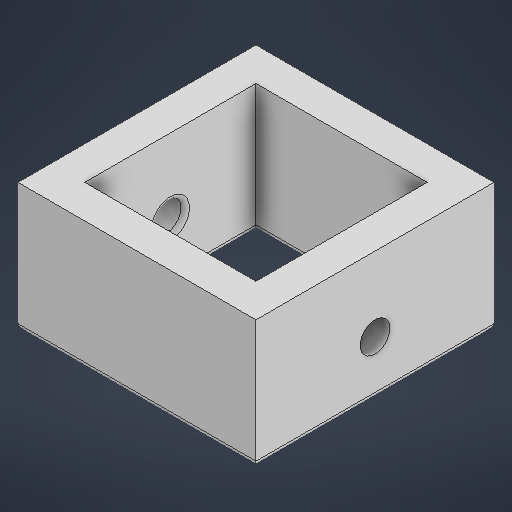
# Autodesk Inventor part: TestSujetaPerfil
Saved by Autodesk Inventor 2026.1 (Build 301233020, 233B)
## iProperties
Created: 2025-10-19
Part Number: TestSujetaPerfil
Material: Generic
Document SubType Name: Modeling
Designer: tito.luyo
Density: 1 g/cm^3
Appearance: Default
Author: tito.luyo
Autodesk Inventor part; units mm, degrees
ref_plane "YZ Plane" through (0, 0, 0) normal (1, 0, 0) x (0, 1, 0)
ref_plane "XZ Plane" through (0, 0, 0) normal (0, 1, 0) x (-1, 0, 0)
ref_plane "XY Plane" through (0, 0, 0) normal (0, 0, 1) x (1, 0, 0)
sketch "Sketch1" plane through (0, 0, 0) normal (0, 1, 0) x (-1, 0, 0)
  line L0 (0, 0) -> (28, 0)
  line L1 (28, 0) -> (28, -28)
  line L2 (28, -28) -> (0, -28)
  line L3 (0, -28) -> (0, 0)
  line L4 (24.075, -3.925) -> (3.925, -3.925)
  line L5 (3.925, -3.925) -> (3.925, -24.075)
  line L6 (3.925, -24.075) -> (24.075, -24.075)
  line L7 (24.075, -24.075) -> (24.075, -3.925)
  line L8 (24.075, -3.925) -> (3.925, -24.075) construction
  line L9 (3.925, -3.925) -> (24.075, -24.075) construction
  line L10 (0, 0) -> (28, -28) construction
  line L11 (28, 0) -> (0, -28) construction
  point P0 (14, -14)
  dimension "d0" = 28
  dimension "d1" = 28
  dimension "d2" = 20.15
  dimension "d3" = 20.15
  constraints: 24 end point, 4 parallel, 3 midpoint, 2 horizontal, 2 perpendicular
  measures "d0" distance of L1.end L2.end
  measures "d1" distance of L0.end L1.end
  measures "d2" distance of L6.end L5.end
  measures "d3" distance of L5.end L4.end
extrude "Extrusion1" add sketch "Sketch1" along normal blind 15
fillet "Fillet1" radius 0.6 8 edges at (-14, 0, -3.925) (-24.075, 0, -14) (-14, 0, -24.075) (-3.925, 0, -14) (-14, 0, 0) (-28, 0, -14) (-14, 0, -28) (0, 0, -14)
sketch "Sketch2" plane through (-28, 15, -28) normal (-1, 0, 0) x (0, 0, 1)
  circle A0 centre (14, -8.7403) radius 1.75
  point P0 (28, -15)
  dimension "d7" = 3.5
  constraints: 1 centre point
  measures "d7" diameter of A0
extrude "Extrusion2" cut sketch "Sketch2" against normal blind 10
sketch "Sketch3" plane through (0, 15, 0) normal (1, 0, 0) x (0, 0, -1)
  circle A0 centre (14, -8.7403) radius 1.75 projected
  circle A1 centre (14, -8.7403) radius 1.75
  point P0 (0, -15)
  dimension "d10" = 3.5
  constraints: 1 centre point, 1 coincident
  measures "d10" diameter of A1
extrude "Extrusion3" cut sketch "Sketch3" against normal blind 10
fillet "Fillet2" radius 0.5 2 edges at (-3.925, 6.2597, -12.25) (-24.075, 6.2597, -15.75)
body "Solid1"
